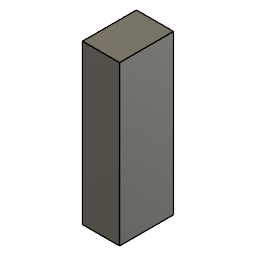
bus+bar+mock (Autodesk Fusion 360 design; units mm, degrees)
part number: 2026-02-08-16-14-46-346
Autodesk Fusion 360 part; units mm, degrees
sketch "Sketch1" plane through (0, 0, 0) normal (0, 0, 1) x (1, 0, 0)
  line L0 (-34.3354, 29.5736) -> (0.5896, 29.5736)
  line L1 (0.5896, 29.5736) -> (0.5896, -119.6514)
  line L2 (0.5896, -119.6514) -> (-34.3354, -119.6514)
  line L3 (-34.3354, -119.6514) -> (-34.3354, 29.5736)
  dimension "d1" = 34.925
  dimension "d2" = 149.225
  constraint horizontal L0
  constraint vertical L1
  constraint horizontal L2
  constraint vertical L3
  measures "d1" distance of L0.start L0.end
  measures "d2" distance of L0.start L2.end
extrude "Extrude1" add sketch "Sketch1" along normal blind 50.8
